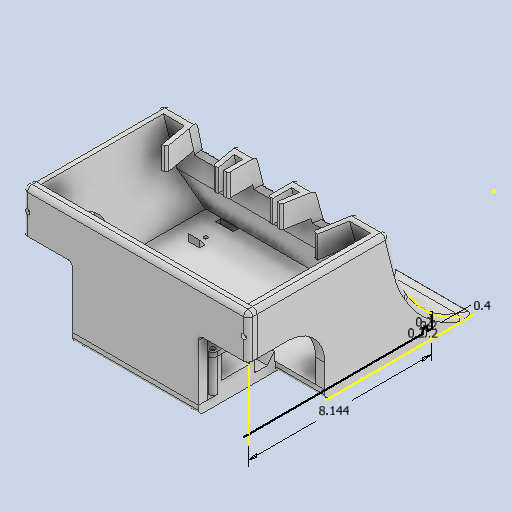
# Autodesk Inventor part: Body
Saved by Autodesk Inventor 2024 (Build 280153000, 153)
## iProperties
Created: 2023-10-20
Part Number: Body
Material: Generic
Document SubType Name: Modeling
Designer: kdcao
Density: 1 g/cm^3
Appearance: Default
Mass: 95.0467 g
Surface Area: 549.579 cm^2
Volume: 95.0467 cm^3
Author: kdcao
Autodesk Inventor part; units mm, degrees
ref_plane "YZ Plane" through (0, 0, 0) normal (1, 0, 0) x (0, 1, 0)
ref_plane "XZ Plane" through (0, 0, 0) normal (0, 1, 0) x (-1, 0, 0)
ref_plane "XY Plane" through (0, 0, 0) normal (0, 0, 1) x (1, 0, 0)
sketch "Sketch1" plane through (0, 0, 0) normal (0, 1, 0) x (-1, 0, 0)
  line L0 (-50, 50) -> (50, 50)
  line L1 (50, 50) -> (50, -50)
  line L2 (50, -50) -> (-50, -50)
  line L3 (-50, -50) -> (-50, 50)
  line L4 (-50, 50) -> (50, -50) construction
  line L5 (50, 50) -> (-50, -50) construction
  point P0 (0, 0)
  dimension "d0" = 100
  dimension "d1" = 100
  constraints: 12 end point, 2 midpoint, 2 parallel, 1 horizontal, 1 perpendicular
  measures "d0" distance of L0.end L1.end
  measures "d1" distance of L1.end L2.end
extrude "Extrusion1" add sketch "Sketch1" along normal blind 50
sketch "Sketch2" plane through (50, 0, 50) normal (1, 0, 0) x (0, 0, -1)
  line L0 (100, 0) -> (100, 50)
  line L1 (100, 0.1) -> (79.65571, 7.504716)
  line L2 (79.65571, 7.504716) -> (68.108704, 27.504716)
  line L3 (100, 50) -> (0, 50)
  line L4 (100, 50) -> (100, 0.1)
  line L5 (0, 0) -> (100, 0)
  line L6 (62.5, 50) -> (68.108704, 27.504716)
  point P0 (50, 0)
  dimension "d4" = 20
  dimension "d5" = 60
  dimension "d6" = 0.1
  dimension "d18" = 62.5
  dimension "d19" = 76
  dimension "d20" = 20
  constraints: 8 end point, 2 point on line, 1 vertical
  measures "d4" angle of L5 L1
  measures "d5" angle of L3 L2
  measures "d6" distance of L0.start L1.start
  measures "d18" distance of L6.start L3.end
  measures "d19" angle of L6 L3
  measures "d20" vertical distance of L1.end L2.end
extrude "Extrusion2" cut sketch "Sketch2" against normal through all
shell "Shell1" thickness 3.999992 removed faces 1 at (16.666667, 50, 29.166667)
sketch "Sketch3" plane through (50, 0, 50) normal (1, 0, 0) x (0, 0, -1)
  circle A0 centre (17.5, 14.5) radius 16.5
  line L0 (0, 0) -> (0, 50)
  line L1 (0, 0) -> (100, 0)
  line L2 (0, 14.5) -> (0, 0)
  line L3 (0, 0) -> (34, 0)
  line L4 (34, 14.5) -> (34, 0)
  line L5 (91.343613, 1.5748) -> (0, 1.5748)
  line L6 (17.5, 31) -> (0, 31)
  point P0 (50, 0)
  point P1 (98.4125, 1.5875)
  point P2 (0, 1.5748)
  point P3 (91.271588, 1.5875)
  dimension "d12" = 33
  dimension "d13" = 17.5
  dimension "d14" = 14.5
  constraints: 8 end point, 2 point on circle, 2 point on line, 1 centre point, 1 collinear, 1 perpendicular, 1 tangent, 1 vertical, 1 other
  measures "d12" diameter of A0
  measures "d13" distance from line of L0 A0.centre
  measures "d14" distance from line of L1 A0.centre
extrude "Extrusion3" cut sketch "Sketch3" against normal blind 22 contours A0 L5 | L4 L5 A0 | A0 L5 L0 L6 | L5 L4 L1 A0 | A0 L1 L5 | A0 L1 L0 L5
ref_plane "Work Plane1" through (0, 0, -50) normal (1, 0, 0) x (0, 0, -1)
mirror "Mirror1" about plane through (0, 0, -50) normal (1, 0, 0) of "Extrusion3"
fillet "Fillet1" radius 43.275 1 edges at (0, 7.5047, -29.6557)
fillet "Fillet2" radius 40 1 edges at (0, 27.5047, -18.1087)
sketch "Sketch27" plane through (-50, 50, 50) normal (0, 0, 1) x (1, 0, 0)
  line L0 (0, -19) -> (0, 0) projected
  line L1 (100, -19) -> (100, 0) projected
  point P0 (50, -50)
  point P1 (2, -9.5)
  point P2 (98, -9.5)
  point P3 (0, -9.5)
  point P4 (100, -9.5)
  dimension "d156" = 2
  dimension "d157" = 0
  dimension "d158" = 2
  dimension "d159" = 0
  constraints: 2 midpoint
  measures "d156" distance from line of L0 point (2, -9.5)
  measures "d157" vertical distance of point (0, -9.5) point (2, -9.5)
  measures "d158" distance from line of L1 point (98, -9.5)
  measures "d159" vertical distance of point (100, -9.5) point (98, -9.5)
hole "Hole5" at (-48, 40.5, 50) at (48, 40.5, 50) direction (0, 0, -1) diameter 1.75 depth 5.83 counterbore diameter 2.2 counterbore depth 1.2
sketch "Sketch28" plane through (0, 0, 0) normal (0, -1, 0) x (1, 0, 0)
  line L0 (-28, 50) -> (28, 50) projected
  line L1 (28, 16) -> (28, 50) projected
  line L2 (-28, 50) -> (-28, 16) projected
  line L3 (-50, -50) -> (-50, 16) projected
  line L4 (-28, 16) -> (-50, 16) projected
  line L5 (50, 16) -> (28, 16) projected
  line L6 (50, 16) -> (50, -50) projected
  point P0 (0, 0)
  point P1 (-24, 48)
  point P2 (24, 48)
  point P3 (-48, 12)
  point P4 (48, 12)
  dimension "d160" = 2
  dimension "d161" = 2
  dimension "d162" = 4
  dimension "d163" = 4
  dimension "d164" = 2
  dimension "d165" = 4
  dimension "d166" = 4
  dimension "d167" = 2
  measures "d160" distance from line of L0 point (-24, 48)
  measures "d161" distance from line of L0 point (24, 48)
  measures "d162" distance from line of L1 point (24, 48)
  measures "d163" distance from line of L2 point (-24, 48)
  measures "d164" distance from line of L3 point (-48, 12)
  measures "d165" distance from line of L4 point (-48, 12)
  measures "d166" distance from line of L5 point (48, 12)
  measures "d167" distance from line of L6 point (48, 12)
hole "Hole6" at (-24, 0, 48) at (24, 0, 48) at (-48, 0, 12) at (48, 0, 12) direction (0, 1, 0) diameter 1.75 depth 5.83 counterbore diameter 2.2 counterbore depth 1.2
sketch "Sketch4" plane through (50, 50, 50) normal (1, 0, 0) x (0, 0, -1)
  line L0 (-2.216786, -46.000008) -> (77.440919, -46.000008)
  arc A0 (71.780304, -28.854681) -> (94.456631, -47.882379) centre (109.257553, -7.217181) ccw
  line L1 (34, -50) -> (100, -50)
  line L2 (77.440919, -46.000008) -> (77.440919, -44.000008)
  line L3 (77.440919, -44.000008) -> (79.440919, -44.000008)
  line L4 (79.440919, -46.000008) -> (81.440919, -46.000008)
  line L5 (81.440919, -40.344966) -> (81.440919, -40.367754)
  line L6 (79.440919, -44.000008) -> (79.440919, -46.000008)
  line L7 (81.440919, -46.000008) -> (81.440919, -40.367754)
  line L8 (0, -50) -> (0, -19)
  point P0 (50, -50)
  dimension "d73" = 2
  dimension "d75" = 3.99999
  dimension "d76" = 2
  dimension "d77" = 2
  dimension "d78" = 2
  dimension "d79" = 81.44092
  constraints: 14 end point, 3 perpendicular, 3 point on circle, 2 vertical, 1 horizontal
  measures "d73" distance of L2.end L3.end
  measures "d75" distance between parallel lines of L1 L0
  measures "d76" distance of L0.end L2.end
  measures "d77" distance of L3.end L4.start
  measures "d78" distance of L4.start L4.end
  measures "d79" distance from line of L8 L4.end
split body "Split1" sketch "Sketch4" result two bodies curves L0 L2 L3 L6 L4 L7 first body at (-9.333333, 43.666667, 49.5)
sketch "Sketch5" plane through (-50, 0, -50) normal (-1, 0, 0) x (0, 0, 1)
  line L0 (66, 3.999992) -> (22.559081, 3.999992)
  line L1 (39.2, 3.999992) -> (39.2, 6.999992)
  line L2 (39.2, 6.999992) -> (36.856143, 3.999992)
  line L3 (36.856143, 3.999992) -> (39.2, 3.999992)
  line L4 (100, 3.999992) -> (100, 0)
  line L5 (66, 0) -> (66, 3.999992)
  point P0 (50, 0)
  point P1 (17.410334, 3.999992)
  dimension "d28" = 3
  dimension "d29" = 38
  dimension "d43" = 26.8
  constraints: 6 end point, 2 perpendicular, 1 point on line
  measures "d28" distance of L1.start L1.end
  measures "d29" angle of L1 L2
  measures "d43" distance from line of L1.start L5
ref_plane "Work Plane2" through (-37.5, 0, -50) normal (-1, 0, 0) x (0, 0, 1)
extrude "Extrusion4" add sketch "Sketch5" against normal blind 5.15 from surface at -12.5 bodies 3
sketch "Sketch6" plane through (-28, 0, 16) normal (-1, 0, 0) x (0, 0, 1)
  line L0 (34, 3.999992) -> (0, 3.999992)
  line L1 (7.3, 3.999992) -> (7.3, 18.599992)
  line L2 (7.3, 18.599992) -> (11.3, 18.599992)
  line L3 (11.3, 18.599992) -> (11.3, 8.499992)
  line L4 (11.3, 8.499992) -> (23.7, 8.499992)
  line L5 (23.7, 8.499992) -> (23.7, 18.599992)
  line L6 (23.7, 18.599992) -> (27.7, 18.599992)
  line L7 (27.7, 18.599992) -> (27.7, 3.999992)
  line L8 (7.3, 3.999992) -> (27.7, 3.999992)
  line L9 (34, 3.999992) -> (34, 0)
  line L10 (7.3, 18.599992) -> (27.7, 18.599992)
  line L11 (27.7, 18.599992) -> (27.7, 20.599992)
  line L12 (27.7, 20.599992) -> (7.3, 20.599992)
  line L13 (7.3, 20.599992) -> (7.3, 18.599992)
  point P0 (-16, 0)
  point P1 (27.7, 18.599992)
  dimension "d34" = 12.4
  dimension "d38" = 4
  dimension "d39" = 4
  dimension "d40" = 10.3
  dimension "d168" = 10.1
  dimension "d169" = 14.6
  dimension "d170" = 2
  dimension "d171" = 20.4
  constraints: 24 end point, 7 perpendicular, 4 point on line, 2 parallel, 1 collinear, 1 horizontal
  measures "d34" distance of L3.end L4.end
  measures "d38" distance of L5.end L6.end
  measures "d39" distance of L1.end L2.end
  measures "d40" distance between parallel lines of L9 L5
  measures "d168" distance of L2.end L3.end
  measures "d169" distance of L6.end L7.end
  measures "d170" distance of L12.end L1.end
  measures "d171" distance of L11.end L12.end
extrude "Extrusion5" add sketch "Sketch6" against normal blind 25.7875 contours L0 L1 L2 L3 L4 L5 L6 L7 | L6 L10 L2 L13 L12 L11 bodies 3
mirror "Mirror2" about plane through (0, 0, -50) normal (1, 0, 0) of "Extrusion5", "Extrusion4" bodies 3
sketch "Sketch7" plane through (-28, 0, 16) normal (-1, 0, 0) x (0, 0, 1)
  line L0 (34, 3.999992) -> (0, 3.999992)
  line L1 (0.4, 3.999992) -> (0.4, 7.999992)
  line L2 (0.4, 7.999992) -> (3.4, 3.999992)
  line L3 (0, 0) -> (0, 3.999992)
  point P0 (-16, 0)
  point P1 (7.3, 3.999992)
  dimension "d44" = 0.4
  dimension "d45" = 3
  dimension "d46" = 4
  constraints: 4 end point, 2 point on line, 1 perpendicular
  measures "d44" distance from line of L3 L1.start
  measures "d45" distance from line of L2.end L1
  measures "d46" distance of L1.start L1.end
extrude "Extrusion6" add sketch "Sketch7" against normal blind 5.15 bodies 3
mirror "Mirror3" about plane through (0, 0, -50) normal (1, 0, 0) of "Extrusion6" bodies 3
sketch "Sketch9" plane through (28, 3.999992, 16) normal (0, 1, 0) x (1, 0, 0)
  line L0 (-66.85, 42.8) -> (-59.15, 42.8)
  line L1 (-59.15, 42.8) -> (-59.15, 30)
  line L2 (-59.15, 30) -> (-66.85, 30)
  line L3 (-66.85, 30) -> (-66.85, 42.8)
  line L4 (-66.85, 42.8) -> (-59.15, 30) construction
  line L5 (-59.15, 42.8) -> (-66.85, 30) construction
  line L6 (-78, 0) -> (-78, 43.440919)
  line L7 (-78, 0) -> (-56, 0)
  point P0 (-28, 16)
  point P1 (-63, 36.4)
  point P2 (-78, 48.589666)
  point P3 (-63, 30)
  dimension "d49" = 12.8
  dimension "d50" = 7.7
  dimension "d51" = 15
  dimension "d52" = 30
  constraints: 12 end point, 3 midpoint, 2 parallel, 1 horizontal, 1 perpendicular
  measures "d49" distance of L2.end L0.start
  measures "d50" distance of L1.end L2.end
  measures "d51" distance from line of L6 point (-63, 30)
  measures "d52" distance between parallel lines of L7 L2
extrude "Extrusion7" cut sketch "Sketch9" along normal blind 3 from surface at -3.999992 bodies 3
mirror "Mirror4" about plane through (0, 0, -50) normal (1, 0, 0) of "Extrusion7" bodies 3
ref_plane "Work Plane4" through (-50, 50, -10.5) normal (0, 0, 1) x (1, 0, 0)
sketch "Sketch12" plane through (-50, 50, -10.5) normal (0, 0, 1) x (1, 0, 0)
  line L0 (50.058624, -12.012671) -> (41.208624, -12.012671)
  line L1 (41.208624, -12.012671) -> (41.208624, 0.587329)
  line L2 (41.208624, 0.587329) -> (58.908624, 0.587329)
  line L3 (58.908624, 0.587329) -> (58.908624, -12.012671)
  line L4 (58.908624, -12.012671) -> (50.058624, -12.012671)
  point P0 (50, -50)
  dimension "d61" = 12.6
  dimension "d62" = 17.7
  constraints: 10 end point, 4 perpendicular, 1 collinear, 1 horizontal, 1 point on line
  measures "d61" distance of L2.end L3.end
  measures "d62" distance of L1.end L2.end
extrude "Extrusion9" cut sketch "Sketch12" along normal mid plane 14.7625 bodies 2
ref_plane "Work Plane5" through (34.428051, 50.599992, -7.426419) normal (0.1736482, 0, -0.9848078) x (0, -1, 0)
sketch "Sketch13" plane through (34.428051, 50.599992, -7.426419) normal (0.1736482, 0, -0.9848078) x (0, -1, 0)
  line L0 (0.019911, -0.003019) -> (12.619911, -0.003019)
  line L1 (12.619911, -0.003019) -> (12.619911, 17.696981)
  line L2 (12.619911, 17.696981) -> (0.019911, 17.696981)
  line L3 (0.019911, 17.696981) -> (0.019911, -0.003019)
  point P0 (50.599992, 32.615428)
  dimension "d65" = 17.7
  dimension "d66" = 12.6
  constraints: 8 end point, 2 parallel, 1 horizontal, 1 perpendicular, 1 other
  measures "d65" distance of L2.end L0.start
  measures "d66" distance of L1.end L2.end
extrude "Extrusion10" cut sketch "Sketch13" along normal mid plane 20 bodies 2
ref_plane "Work Plane6" through (-34.428051, 37.999992, -7.426427) normal (0.1736482, 0, 0.9848078) x (0, 1, 0)
sketch "Sketch14" plane through (-34.428051, 37.999992, -7.426427) normal (0.1736482, 0, 0.9848078) x (0, 1, 0)
  line L0 (0, 0) -> (12.6, 0)
  line L1 (12.6, 0) -> (12.6, -17.7)
  line L2 (12.6, -17.7) -> (0, -17.7)
  line L3 (0, -17.7) -> (0, 0)
  point P0 (-37.999992, -32.615426)
  dimension "d69" = 17.7
  dimension "d70" = 12.6
  constraints: 8 end point, 2 parallel, 1 horizontal, 1 perpendicular, 1 other
  measures "d69" distance of L0.end L1.end
  measures "d70" distance of L1.end L2.end
extrude "Extrusion11" cut sketch "Sketch14" along normal mid plane 20 bodies 2
sketch "Sketch15" plane through (0, 0, 0) normal (0, -1, 0) x (1, 0, 0)
  line L0 (31.15, -26.8) -> (31.15, -14)
  line L1 (38.85, -26.8) -> (31.15, -26.8)
  line L2 (31.15, -24.5) -> (38.85, -24.5)
  line L3 (38.85, -24.5) -> (38.85, -26.8)
  line L4 (38.85, -26.8) -> (31.15, -26.8)
  line L5 (31.15, -26.8) -> (31.15, -24.5)
  circle A0 centre (35, -16.15079) radius 0.875
  line L6 (50, 16) -> (50, -50)
  line L7 (50, -50) -> (-50, -50)
  point P0 (0, 0)
  dimension "d80" = 15
  dimension "d81" = 1.75
  dimension "d82" = 2.3
  dimension "d83" = 33.84921
  constraints: 8 end point, 2 parallel, 1 centre point, 1 horizontal, 1 perpendicular, 1 point on line
  measures "d80" distance from line of L6 A0.centre
  measures "d81" diameter of A0
  measures "d82" distance of L2.end L1.start
  measures "d83" distance from line of L7 A0.centre
extrude "Extrusion12" cut sketch "Sketch15" against normal through all bodies 3
mirror "Mirror5" about plane through (0, 0, -50) normal (1, 0, 0) of "Extrusion12" bodies 3
sketch "Sketch16" plane through (50, 50, 50) normal (1, 0, 0) x (0, 0, -1)
  line L0 (4, -20.780502) -> (4, 0)
  line L1 (0, -19) -> (0, 0)
  point P0 (50, -50)
  dimension "d86" = 4
  constraints: 2 end point
  measures "d86" distance between parallel lines of L1 L0
split body "Split2" sketch "Sketch16" result two bodies bodies 2 curves L0 first body at (-9.333333, 43.666667, 49.5)
sketch "Sketch17" plane through (0, 50, 0) normal (0, 1, 0) x (1, 0, 0)
  line L0 (35.85416, 15.496902) -> (35.325726, 12.5)
  line L1 (35.325726, 12.5) -> (32.504494, -3.5)
  line L2 (32.504494, -3.5) -> (34.504494, -3.852654)
  line L3 (34.504494, -3.852654) -> (37.325726, 12.147346)
  line L4 (37.325726, 12.147346) -> (35.325726, 12.5)
  line L5 (17.352674, 12.5) -> (8.908624, 12.5)
  line L6 (17.352674, 12.5) -> (15.060424, -0.5)
  line L7 (15.060424, -0.5) -> (13.060424, -0.147346)
  line L8 (13.060424, -0.147346) -> (15.290492, 12.5)
  line L9 (17.352674, 12.5) -> (15.290492, 12.5)
  point P0 (0, 0)
  dimension "d87" = 2
  dimension "d88" = 16
  dimension "d89" = 2
  dimension "d93" = 12.64735
  constraints: 16 end point, 3 parallel, 2 perpendicular, 1 collinear, 1 point on line
  measures "d87" horizontal distance of L1.end L2.end
  measures "d88" vertical distance of L2.end L3.end
  measures "d89" horizontal distance of L6.end L7.end
  measures "d93" vertical distance of L7.end L8.end
extrude "Extrusion13" add sketch "Sketch17" against normal blind 10 bodies 5
mirror "Mirror6" about plane through (0, 0, -50) normal (1, 0, 0) of "Extrusion13" bodies 5
sketch "Sketch18" plane through (0, 50, 0) normal (0, 1, 0) x (1, 0, 0)
  line L0 (17.352674, 12.5) -> (8.908624, 12.5)
  line L1 (8.908624, 12.5) -> (8.908624, 0)
  line L2 (8.908624, 0) -> (10.908624, 0)
  line L3 (10.908624, 0) -> (10.908624, 12.5)
  line L4 (10.908624, 12.5) -> (8.908624, 12.5)
  line L5 (-8.791376, 15.495095) -> (-8.791376, 11.372649)
  line L6 (-8.791376, 12.5) -> (-8.791376, 0)
  line L7 (-8.791376, 0) -> (-10.791376, 0)
  line L8 (-10.791376, 0) -> (-10.791376, 12.5)
  line L9 (-10.791376, 12.5) -> (-8.791376, 12.5)
  point P0 (0, 0)
  dimension "d94" = 2
  dimension "d95" = 2
  dimension "d96" = 12.5
  constraints: 16 end point, 4 parallel, 3 perpendicular, 3 point on line, 1 collinear
  measures "d94" distance of L1.end L2.end
  measures "d95" distance of L6.end L7.end
  measures "d96" distance of L2.end L3.end
extrude "Extrusion14" add sketch "Sketch18" against normal blind 10 bodies 5
sketch "Sketch31" plane through (-28, 20.599992, 43.7) normal (0, 1, 0) x (1, 0, 0)
  line L0 (0, 20.4) -> (25.7875, 20.4) projected
  line L1 (25.7875, 20.4) -> (25.7875, 0) projected
  line L2 (0, 0) -> (25.7875, 0) projected
  line L3 (0, 0) -> (0, 20.4) projected
  point P0 (28, 43.7)
  point P1 (23.7875, 18.4)
  point P2 (23.7875, 2)
  point P3 (2, 2)
  point P4 (2, 18.4)
  dimension "d180" = 2
  dimension "d181" = 2
  dimension "d182" = 2
  dimension "d183" = 2
  dimension "d184" = 2
  dimension "d185" = 2
  dimension "d186" = 2
  dimension "d187" = 2
  measures "d180" distance from line of L0 point (23.787, 18.4)
  measures "d181" distance from line of L1 point (23.787, 18.4)
  measures "d182" distance from line of L1 point (23.787, 2)
  measures "d183" distance from line of L2 point (23.787, 2)
  measures "d184" distance from line of L2 point (2, 2)
  measures "d185" distance from line of L3 point (2, 2)
  measures "d186" distance from line of L0 point (2, 18.4)
  measures "d187" distance from line of L3 point (2, 18.4)
hole "Hole7" at (-4.2125, 20.599992, 25.3) at (-4.2125, 20.599992, 41.7) at (-26, 20.599992, 41.7) at (-26, 20.599992, 25.3) direction (0, -1, 0) diameter 1.75 depth 5.83 counterbore diameter 2.2 counterbore depth 1.2 bodies 3
mirror "Mirror7" about plane through (0, 0, -50) normal (1, 0, 0) of "Hole7" bodies 3
sketch "Sketch32" plane through (-28, 0, 16) normal (-1, 0, 0) x (0, 0, 1)
  line L0 (7.3, 3.999992) -> (7.3, 20.599992)
  line L1 (7.3, 18.599992) -> (27.7, 18.599992)
  line L2 (27.7, 20.599992) -> (27.7, 3.999992)
  point P0 (-16, 0)
  point P1 (11.3, 18.599992)
  constraints: 3 point on line, 2 end point, 1 horizontal
split body "Split6" sketch "Sketch32" result two bodies bodies 3 curves L1 first body at (11.776761, 20.099992, 36.025043) (-11.776761, 20.099992, 36.025043)
fillet "Fillet3" radius 2 28 edges at (-50, 40.5, 50) (-50, 50, 48) (0, 50, 50) (50, 50, 48) (50, 40.5, 50) (-28, 31, 48) (28, 31, 48) (-50, 50, 16.75) (-42.6613, 50, -12.5) (-50, 27.652, -18.4732) (-50, 21.8908, -21.3499) (-50, 14.9662, -26.107) (-50, 41.4797, -14.6244) (-13.0705, 50, -12.5) (13.1306, 50, -12.5) (42.6629, 50, -12.5) (50, 27.652, -18.4732) (50, 21.8908, -21.3499) (50, 14.9662, -26.107) (50, 41.4797, -14.6244) (50, 50, 16.75) (-50, 1.1088, -47.2283) (-50, 5.3056, -37.6201) (50, 1.1088, -47.2283) (50, 5.3056, -37.6201) (0, 0, 50) (39, 0, 16) (-39, 0, 16)
fillet "Fillet4" radius 2 8 edges at (-28, 19.6, 43.7) (-28, 19.6, 23.3) (-2.2125, 19.6, 23.3) (-2.2125, 19.6, 43.7) (-28, 11.3, 43.7) (-28, 11.3, 23.3) (-2.2125, 11.3, 23.3) (-2.2125, 11.3, 43.7)
fillet "Fillet5" radius 1 6 edges at (32.5045, 45, 3.5) (15.0604, 45, 0.5) (8.9086, 45, 0) (-8.7914, 45, 0) (-15.0604, 45, 0.5) (-32.5045, 45, 3.5)
fillet "Fillet6" radius 1 3 edges at (-26.8637, 38, -15.4919) (0.0586, 37.9873, -15.4951) (26.8676, 37.9801, -15.4969)
mirror "Mirror8" about plane through (0, 0, -50) normal (1, 0, 0) of "Fillet4"
body "Solid4"
body "Solid5"
body "Solid12"
body "Solid13"
